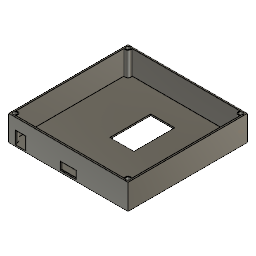
incubetter base (Autodesk Fusion 360 design; units mm, degrees)
Autodesk Fusion 360 part; units mm, degrees
sketch "Sketch1" plane through (0, 0, 0) normal (0, 0, 1) x (1, 0, 0)
  line L0 (75, -75) -> (-75, -75)
  line L1 (-75, -75) -> (-75, 75)
  line L2 (-75, 75) -> (75, 75)
  line L3 (75, 75) -> (75, -75)
  line L4 (75, -75) -> (-75, 75) construction
  line L5 (-75, -75) -> (75, 75) construction
  dimension "d1" = 150
  dimension "d2" = 150
extrude "Extrude1" add sketch "Sketch1" along normal blind 2
sketch "Sketch2" plane through (0, 0, 2) normal (0, 0, 1) x (-1, 0, 0)
  line L0 (-75, -75) -> (75, -75)
  line L1 (75, -75) -> (75, 75)
  line L2 (75, 75) -> (-75, 75)
  line L3 (-75, 75) -> (-75, -75)
  line L4 (75, -75) -> (73, -75)
  line L5 (73, -75) -> (73, 75)
  line L6 (73, 75) -> (75, 75)
  line L7 (75, 75) -> (75, -75)
extrude "Extrude2" add sketch "Sketch2" along normal blind 30 contours L0 L1 L2 L4 L5 L6 L7
sketch "Sketch3" plane through (0, 0, 2) normal (0, 0, 1) x (-1, 0, 0)
  line L0 (73, -75) -> (73, 75)
  line L1 (73, 75) -> (-75, 75)
  line L2 (-75, 75) -> (-75, -75)
  line L3 (-75, -75) -> (73, -75)
  line L4 (73, -75) -> (-75, -75)
  line L5 (-75, -75) -> (-75, -73)
  line L6 (-75, -73) -> (73, -73)
  line L7 (73, -73) -> (73, -75)
extrude "Extrude3" add sketch "Sketch3" along normal blind 30 contours L0 L2 L3 L4 L5 L6 L7
sketch "Sketch4" plane through (0, 0, 2) normal (0, 0, 1) x (-1, 0, 0)
  line L0 (-75, -73) -> (73, -73)
  line L1 (73, -73) -> (73, 75)
  line L2 (73, 75) -> (-75, 75)
  line L3 (-75, 75) -> (-75, -73)
  line L4 (-75, -73) -> (-73, -73)
  line L5 (-73, -73) -> (-73, 75)
  line L6 (-73, 75) -> (-75, 75)
  line L7 (-75, 75) -> (-75, -73)
  dimension "d9" = 2
  dimension "d10" = 148
extrude "Extrude4" add sketch "Sketch4" along normal blind 30 contours L0 L2 L3 L4 L5 L6 L7
sketch "Sketch5" plane through (0, 0, 2) normal (0, 0, 1) x (-1, 0, 0)
  line L0 (-73, 75) -> (-73, -73)
  line L1 (-73, -73) -> (73, -73)
  line L2 (73, -73) -> (73, 75)
  line L3 (73, 75) -> (-73, 75)
  line L4 (0, 0) -> (0, -18)
  line L5 (-15, 7.5) -> (15, 7.5)
  line L6 (15, 7.5) -> (15, -43.5)
  line L7 (15, -43.5) -> (-15, -43.5)
  line L8 (-15, -43.5) -> (-15, 7.5)
  line L9 (-15, 7.5) -> (15, -43.5) construction
  line L10 (15, 7.5) -> (-15, -43.5) construction
  dimension "d13" = 18
  dimension "d14" = 51
  dimension "d15" = 30
  measures "d13" distance of L4.start
extrude "Extrude5" cut sketch "Sketch5" against normal blind 2 contours L5 L6 L7 L8
sketch "Sketch6" plane through (0, 0, 2) normal (0, 0, 1) x (-1, 0, 0)
  line L0 (15, 7.5) -> (15, -43.5)
  line L1 (15, -43.5) -> (-15, -43.5)
  line L2 (-15, -43.5) -> (-15, 7.5)
  line L3 (-15, 7.5) -> (15, 7.5)
  line L4 (-73, 75) -> (-73, -73)
  line L5 (-73, -73) -> (73, -73)
  line L6 (73, -73) -> (73, 75)
  line L7 (73, 75) -> (-73, 75)
  line L8 (-73, 75) -> (73, 75)
  line L9 (73, 75) -> (73, 73)
  line L10 (73, 73) -> (-73, 73)
  line L11 (-73, 73) -> (-73, 75)
extrude "Extrude6" add sketch "Sketch6" along normal blind 30 contours L4 L6 L7 L8 L9 L10 L11
sketch "Sketch7" plane through (0, -75, 0) normal (0, -1, 0) x (1, 0, 0)
  line L0 (-75, 0) -> (75, 0)
  line L1 (75, 0) -> (75, 32)
  line L2 (75, 32) -> (-75, 32)
  line L3 (-75, 32) -> (-75, 0)
  line L4 (0, 0) -> (0, 4.8857)
  line L5 (0, 4.8857) -> (0, 9.8857)
  line L6 (0, 9.8857) -> (0, 7.3857)
  line L7 (10, 12.3857) -> (-10, 12.3857)
  line L8 (-10, 12.3857) -> (-10, 2.3857)
  line L9 (-10, 2.3857) -> (10, 2.3857)
  line L10 (10, 2.3857) -> (10, 12.3857)
  line L11 (10, 12.3857) -> (-10, 2.3857) construction
  line L12 (-10, 12.3857) -> (10, 2.3857) construction
  dimension "d20" = 5
  dimension "d21" = 2.5
  dimension "d22" = 20
  dimension "d23" = 10
extrude "Extrude7" cut sketch "Sketch7" against normal blind 4 contours L7 L8 L9 L10
sketch "Sketch8" plane through (0, -75, 0) normal (0, -1, 0) x (1, 0, 0)
  line L0 (-10, 12.3857) -> (10, 12.3857)
  line L1 (10, 12.3857) -> (10, 2.3857)
  line L2 (10, 2.3857) -> (-10, 2.3857)
  line L3 (-10, 2.3857) -> (-10, 12.3857)
  line L4 (-75, 0) -> (75, 0)
  line L5 (75, 0) -> (75, 32)
  line L6 (75, 32) -> (-75, 32)
  line L7 (-75, 32) -> (-75, 0)
  line L8 (-60, 0) -> (-60, 10)
  line L9 (-53.5, 2) -> (-66.5, 2)
  line L10 (-66.5, 2) -> (-66.5, 18)
  line L11 (-66.5, 18) -> (-53.5, 18)
  line L12 (-53.5, 18) -> (-53.5, 2)
  line L13 (-53.5, 2) -> (-66.5, 18) construction
  line L14 (-66.5, 2) -> (-53.5, 18) construction
  dimension "d26" = 13
extrude "Extrude8" cut sketch "Sketch8" against normal blind 4 contours L9 L10 L11 L12
sketch "Sketch9" plane through (0, 0, 2) normal (0, 0, 1) x (-1, 0, 0)
  line L0 (53.5, 73) -> (-73, 73)
  line L1 (-73, 73) -> (-73, -73)
  line L2 (-73, -73) -> (73, -73)
  line L3 (73, -73) -> (73, 73)
  line L4 (73, 73) -> (66.5, 73)
  line L5 (66.5, 73) -> (66.5, 75)
  line L6 (66.5, 75) -> (53.5, 75)
  line L7 (53.5, 75) -> (53.5, 73)
  line L8 (15, 7.5) -> (15, -43.5)
  line L9 (15, -43.5) -> (-15, -43.5)
  line L10 (-15, -43.5) -> (-15, 7.5)
  line L11 (-15, 7.5) -> (15, 7.5)
  circle A0 centre (71, -71) radius 3.5
  dimension "d29" = 7
  measures "d29" diameter of A0
extrude "Extrude9" add sketch "Sketch9" along normal blind 30 contours L2 L3 A0 picked at (70.0212, -70.0212)
sketch "Sketch10" plane through (0, 0, 32) normal (0, 0, 1) x (-1, 0, 0)
  line L0 (73, 73) -> (73, -68.1277)
  arc A0 (73, -68.1277) -> (68.1277, -73) centre (71, -71) ccw
  line L1 (68.1277, -73) -> (-73, -73)
  line L2 (-73, -73) -> (-73, 73)
  line L3 (-73, 73) -> (73, 73)
  line L4 (75, 75) -> (-75, 75)
  line L5 (-75, 75) -> (-75, -75)
  line L6 (-75, -75) -> (75, -75)
  line L7 (75, -75) -> (75, 75)
  circle A1 centre (71, -71) radius 2.5
  dimension "d32" = 5
  measures "d32" diameter of A1
extrude "Extrude10" cut sketch "Sketch10" against normal blind 20 contours A1
sketch "Sketch11" plane through (0, 0, 2) normal (0, 0, 1) x (-1, 0, 0)
  line L0 (15, 7.5) -> (15, -43.5)
  line L1 (15, -43.5) -> (-15, -43.5)
  line L2 (-15, -43.5) -> (-15, 7.5)
  line L3 (-15, 7.5) -> (15, 7.5)
  arc A0 (73, -68.1277) -> (68.1277, -73) centre (71, -71) ccw
  line L4 (73, -68.1277) -> (73, 73)
  line L5 (73, 73) -> (66.5, 73)
  line L6 (66.5, 73) -> (66.5, 75)
  line L7 (66.5, 75) -> (53.5, 75)
  line L8 (53.5, 75) -> (53.5, 73)
  line L9 (53.5, 73) -> (-73, 73)
  line L10 (-73, 73) -> (-73, -73)
  line L11 (-73, -73) -> (68.1277, -73)
  circle A1 centre (-71, -71) radius 3.5
  dimension "d35" = 7
  measures "d35" diameter of A1
extrude "Extrude11" add sketch "Sketch11" along normal blind 30 contours L10 L11 A1 picked at (-70.0436, -69.9989)
sketch "Sketch12" plane through (0, 0, 32) normal (0, 0, 1) x (-1, 0, 0)
  circle A0 centre (71, -71) radius 2.5
  line L0 (73, 73) -> (73, -68.1277)
  arc A1 (73, -68.1277) -> (68.1277, -73) centre (71, -71) ccw
  line L1 (68.1277, -73) -> (-68.1277, -73)
  arc A2 (-68.1277, -73) -> (-73, -68.1277) centre (-71, -71) ccw
  line L2 (-73, -68.1277) -> (-73, 73)
  line L3 (-73, 73) -> (73, 73)
  line L4 (75, 75) -> (-75, 75)
  line L5 (-75, 75) -> (-75, -75)
  line L6 (-75, -75) -> (75, -75)
  line L7 (75, -75) -> (75, 75)
  circle A3 centre (-71, -71) radius 2.5
  dimension "d38" = 5
  measures "d38" diameter of A3
extrude "Extrude12" cut sketch "Sketch12" against normal blind 20 contours A3
sketch "Sketch13" plane through (0, 0, 2) normal (0, 0, 1) x (-1, 0, 0)
  arc A0 (-68.1277, -73) -> (-73, -68.1277) centre (-71, -71) ccw
  line L0 (-68.1277, -73) -> (68.1277, -73)
  arc A1 (73, -68.1277) -> (68.1277, -73) centre (71, -71) ccw
  line L1 (73, -68.1277) -> (73, 73)
  line L2 (73, 73) -> (66.5, 73)
  line L3 (66.5, 73) -> (66.5, 75)
  line L4 (66.5, 75) -> (53.5, 75)
  line L5 (53.5, 75) -> (53.5, 73)
  line L6 (53.5, 73) -> (-73, 73)
  line L7 (-73, 73) -> (-73, -68.1277)
  line L8 (15, 7.5) -> (15, -43.5)
  line L9 (15, -43.5) -> (-15, -43.5)
  line L10 (-15, -43.5) -> (-15, 7.5)
  line L11 (-15, 7.5) -> (15, 7.5)
  circle A2 centre (-71, 71) radius 3.5
  dimension "d41" = 7
  measures "d41" diameter of A2
extrude "Extrude13" add sketch "Sketch13" along normal blind 30 contours L6 L7 A2 picked at (-70.0436, 69.9989)
sketch "Sketch14" plane through (0, 0, 32) normal (0, 0, 1) x (-1, 0, 0)
  circle A0 centre (-71, -71) radius 2.5
  circle A1 centre (71, -71) radius 2.5
  line L0 (73, 73) -> (73, -68.1277)
  arc A2 (73, -68.1277) -> (68.1277, -73) centre (71, -71) ccw
  line L1 (68.1277, -73) -> (-68.1277, -73)
  arc A3 (-68.1277, -73) -> (-73, -68.1277) centre (-71, -71) ccw
  line L2 (-73, -68.1277) -> (-73, 68.1277)
  arc A4 (-73, 68.1277) -> (-68.1277, 73) centre (-71, 71) ccw
  line L3 (-68.1277, 73) -> (73, 73)
  line L4 (75, 75) -> (-75, 75)
  line L5 (-75, 75) -> (-75, -75)
  line L6 (-75, -75) -> (75, -75)
  line L7 (75, -75) -> (75, 75)
  circle A5 centre (-71, 71) radius 2.5
  dimension "d44" = 5
  measures "d44" diameter of A5
extrude "Extrude14" cut sketch "Sketch14" against normal blind 20 contours A5
sketch "Sketch15" plane through (0, 0, 2) normal (0, 0, 1) x (-1, 0, 0)
  line L0 (15, 7.5) -> (15, -43.5)
  line L1 (15, -43.5) -> (-15, -43.5)
  line L2 (-15, -43.5) -> (-15, 7.5)
  line L3 (-15, 7.5) -> (15, 7.5)
  arc A0 (-73, 68.1277) -> (-68.1277, 73) centre (-71, 71) ccw
  line L4 (-73, 68.1277) -> (-73, -68.1277)
  arc A1 (-68.1277, -73) -> (-73, -68.1277) centre (-71, -71) ccw
  line L5 (-68.1277, -73) -> (68.1277, -73)
  arc A2 (73, -68.1277) -> (68.1277, -73) centre (71, -71) ccw
  line L6 (73, -68.1277) -> (73, 73)
  line L7 (73, 73) -> (66.5, 73)
  line L8 (66.5, 73) -> (66.5, 75)
  line L9 (66.5, 75) -> (53.5, 75)
  line L10 (53.5, 75) -> (53.5, 73)
  line L11 (53.5, 73) -> (-68.1277, 73)
  circle A3 centre (71, 71) radius 3.5
  dimension "d47" = 7
  measures "d47" diameter of A3
extrude "Extrude15" add sketch "Sketch15" along normal blind 30 contours L6 L7 A3 picked at (70.0212, 70.0212)
sketch "Sketch16" plane through (0, 0, 32) normal (0, 0, 1) x (-1, 0, 0)
  circle A0 centre (-71, 71) radius 2.5
  circle A1 centre (-71, -71) radius 2.5
  circle A2 centre (71, -71) radius 2.5
  line L0 (73, 68.1277) -> (73, -68.1277)
  arc A3 (73, -68.1277) -> (68.1277, -73) centre (71, -71) ccw
  line L1 (68.1277, -73) -> (-68.1277, -73)
  arc A4 (-68.1277, -73) -> (-73, -68.1277) centre (-71, -71) ccw
  line L2 (-73, -68.1277) -> (-73, 68.1277)
  arc A5 (-73, 68.1277) -> (-68.1277, 73) centre (-71, 71) ccw
  line L3 (-68.1277, 73) -> (68.1277, 73)
  arc A6 (68.1277, 73) -> (73, 68.1277) centre (71, 71) ccw
  line L4 (75, 75) -> (-75, 75)
  line L5 (-75, 75) -> (-75, -75)
  line L6 (-75, -75) -> (75, -75)
  line L7 (75, -75) -> (75, 75)
  circle A7 centre (71, 71) radius 2.5
  dimension "d50" = 5
  measures "d50" diameter of A7
extrude "Extrude16" cut sketch "Sketch16" against normal blind 20 contours A7
sketch "Sketch17" plane through (0, 0, 12) normal (0, 0, 1) x (-1, 0, 0)
  circle A0 centre (-71, -71) radius 2.5
